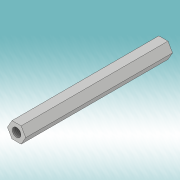
# Autodesk Inventor part: Standoff
Saved by Autodesk Inventor 2019 (Build 230136000, 136)
## iProperties
Created: 2019-01-31
Part Number: Standoff
Material: Generic
Document SubType Name: Modeling
Designer: USUARIO
Density: 1 g/cm^3
Appearance: Default
Author: USUARIO
Autodesk Inventor part; units mm, degrees
ref_plane "YZ Plane" through (0, 0, 0) normal (1, 0, 0) x (0, 1, 0)
ref_plane "XZ Plane" through (0, 0, 0) normal (0, 1, 0) x (-1, 0, 0)
ref_plane "XY Plane" through (0, 0, 0) normal (0, 0, 1) x (1, 0, 0)
sketch "Sketch1" plane through (0, 0, 0) normal (0, 0, 1) x (1, 0, 0)
  line L0 (-1, 1) -> (-4.1754, 1)
  line L1 (-4.1754, 1) -> (-5.7631, 3.75)
  line L2 (-5.7631, 3.75) -> (-4.1754, 6.5)
  line L3 (-4.1754, 6.5) -> (-1, 6.5)
  line L4 (-1, 6.5) -> (0.5877, 3.75)
  line L5 (0.5877, 3.75) -> (-1, 1)
  circle A0 centre (-2.5877, 3.75) radius 2.75
  line L6 (0, -0.1) -> (0, 7.6) projected
  line L7 (-7.0333, 0) -> (1.8579, 0) projected
  circle A1 centre (-2.5877, 3.75) radius 1.5
  dimension "d1" = 5.5
  dimension "d2" = 1
  dimension "d3" = 1
  dimension "d7" = 3
  constraints: 12 end point, 6 tangent, 5 equal length, 2 centre point, 1 coincident, 1 horizontal, 1 parallel
  measures "d1" diameter of A0
  measures "d2" distance from line of L6 L0.start
  measures "d3" distance from line of L7 L0.start
  measures "d7" diameter of A1
extrude "Extrusion1" add sketch "Sketch1" along normal blind 51
thread "Thread3" size "M3x0.5" class "6H" standard "ANSI Metric M Profile" full length
body "Solid1"
